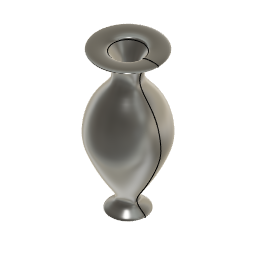
Vase (Autodesk Fusion 360 design; units mm, degrees)
Autodesk Fusion 360 part; units mm, degrees
note: some values were not read from the file. Set by a fixed rule: which sketch regions a step uses.
sketch "Sketch1" plane through (0, 0, 0) normal (0, 1, 0) x (1, 0, 0)
  spline S0 degree 5 poles (14, -101) (13.4463, -100.2053) (12.4158, -98.6486) (11.1003, -96.411) (9.8075, -93.6229) (8.9544, -90.4576) (8.8428, -87.5935) (9.4255, -84.9905) (10.6217, -82.5822) (12.3038, -80.2637) (14.3054, -77.9037) (16.4449, -75.3725) (18.5442, -72.5658) (20.4496, -69.4289) (22.0528, -65.9843) (23.306, -62.3474) (24.2037, -58.68) (24.77, -55.1552) (25.0427, -51.9157) (25.0603, -49.039) (24.8458, -46.4895) (24.399, -44.1084) (23.7064, -41.6855) (22.749, -39.016) (21.5099, -35.9599) (19.9825, -32.5093) (18.1785, -28.7634) (16.137, -24.8872) (13.9324, -21.0763) (11.6845, -17.5192) (9.5646, -14.3622) (7.8104, -11.668) (6.7192, -9.3913) (6.5357, -7.4335) (7.3589, -5.6857) (9.0271, -4.0803) (11.0532, -2.6267) (12.8058, -1.3754) (13.6435, -0.3943) (13.0972, 0.2646) (10.9013, 0.5728) (7.7192, 0.5278) (4.5133, 0.3283) (2.0122, 0.1217) (0.6707, 0) knots 0 0 0 0 0 0 0.025 0.05 0.075 0.1 0.125 0.15 0.175 0.2 0.225 0.25 0.275 0.3 0.325 0.35 0.375 0.4 0.425 0.45 0.475 0.5 0.525 0.55 0.575 0.6 0.625 0.65 0.675 0.7 0.725 0.75 0.775 0.8 0.825 0.85 0.875 0.9 0.925 0.95 0.975 1 1 1 1 1 1
  spline S1 degree 5 poles (11.0799, -103.0346) (11.0751, -103.1807) (11.1108, -103.4624) (11.3005, -103.8539) (11.8276, -104.313) (12.9371, -104.7793) (14.4594, -105.1339) (16.2958, -105.3726) (18.278, -105.492) (20.2008, -105.4886) (21.8446, -105.3598) (23.0026, -105.1037) (23.5039, -104.7199) (23.2473, -104.2115) (22.1889, -103.5831) (20.3196, -102.84) (18.1836, -102.1574) (16.2282, -101.5973) (14.7687, -101.2026) (14, -101) knots 0 0 0 0 0 0 0.066667 0.133333 0.2 0.266667 0.333333 0.4 0.466667 0.533333 0.6 0.666667 0.733333 0.8 0.866667 0.933333 1 1 1 1 1 1
  line L0 (0.6707, 0) -> (0, 0)
  line L1 (0, 0) -> (0.9923, -3.5445)
  spline S2 degree 3 poles (11.0799, -103.0346) (8.564, -99.4237) (6.8311, -96.0686) (5.9843, -92.8003) (5.3345, -90.2929) (5.2446, -87.8077) (5.7478, -85.5198) (6.2508, -83.2327) (7.3186, -81.2184) (8.5491, -79.454) (10.2025, -77.0833) (12.1198, -75.0591) (13.8449, -72.8388) (15.4506, -70.7721) (16.9031, -68.5307) (18.0621, -66.0042) (19.4658, -62.9446) (20.4296, -59.482) (20.9472, -56.2981) (21.3532, -53.8001) (21.4984, -51.5167) (21.4559, -49.6128) (21.4088, -47.4999) (21.1544, -45.8647) (20.6369, -43.9935) (20.1956, -42.3979) (19.5363, -40.5749) (18.6317, -38.3752) (17.4554, -35.5149) (15.8616, -32.035) (13.986, -28.4841) (12.3187, -25.3275) (10.4284, -22.1718) (8.6313, -19.4013) (7.3446, -17.4175) (6.1105, -15.6456) (5.0892, -13.8931) (4.3625, -12.6461) (3.7205, -11.3888) (3.3837, -9.9131) (3.1202, -8.7589) (3.0945, -7.4417) (3.4221, -6.2262) (3.7367, -5.0593) (4.3331, -4.0487) (4.9981, -3.2257) knots 0 0 0 0 0.063857 0.063857 0.063857 0.112846 0.112846 0.112846 0.161819 0.161819 0.161819 0.227618 0.227618 0.227618 0.288865 0.288865 0.288865 0.363038 0.363038 0.363038 0.421232 0.421232 0.421232 0.485816 0.485816 0.485816 0.540886 0.540886 0.540886 0.612496 0.612496 0.612496 0.676153 0.676153 0.676153 0.721732 0.721732 0.721732 0.754166 0.754166 0.754166 0.779534 0.779534 0.779534 0.803888 0.803888 0.803888 0.803888
  spline S3 degree 3 poles (4.9981, -3.2257) (4.2253, -3.2767) (3.3955, -3.3389) (2.5046, -3.4129) (2.0182, -3.4533) (1.514, -3.4972) (0.9923, -3.5445) knots 0.983215 0.983215 0.983215 0.983215 0.994072 0.994072 0.994072 1 1 1 1
  point P0 (10, -84)
  point P1 (25.021, -49.999)
  point P2 (7.3557, -6.0354)
  point P3 (14, -105)
  point P4 (23, -105)
  point P5 (10, -15)
  point P6 (22.5077, -38.4786)
  point P7 (20.0219, -69.9992)
  point P8 (13.019, -0.9995)
  dimension "d1" = -3.559
  constraint coincident L0.end L1.start
  constraint horizontal L0
revolve "Revolve1" add sketch "Sketch1" angle 360 about axis through (0, 0, 1.75) along (0, 0, 1)
named bodies: "Vaza"
